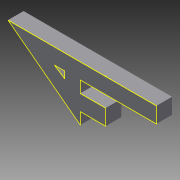
# Autodesk Inventor part: wedger
Saved by Autodesk Inventor 2013 (Build 170138000, 138)
## iProperties
Created: 2013-02-25
Part Number: wedger
Material: Generic
Document SubType Name: Modeling
Designer: Arpan
Density: 1 g/cm^3
Author: Arpan
Autodesk Inventor part; units mm, degrees
ref_plane "YZ Plane" through (0, 0, 0) normal (1, 0, 0) x (0, 1, 0)
ref_plane "XZ Plane" through (0, 0, 0) normal (0, 1, 0) x (-1, 0, 0)
ref_plane "XY Plane" through (0, 0, 0) normal (0, 0, 1) x (1, 0, 0)
sketch "Sketch1" plane through (0, 0, 0) normal (0, 0, 1) x (1, 0, 0)
  line L0 (0, 0) -> (-158.75, 0)
  line L1 (-158.75, 0) -> (-41.275, -88.9)
  line L2 (-41.275, -88.9) -> (-41.275, -25.4)
  line L3 (-41.275, -88.9) -> (-41.275, -69.85)
  line L4 (-41.275, -69.85) -> (0, -69.85)
  line L5 (0, -69.85) -> (0, 0)
  line L6 (-41.275, 0) -> (-66.675, 0)
  line L7 (-66.675, -25.4) -> (-125.1857, -25.4)
  line L8 (-94.622, -48.5293) -> (-79.2945, -28.2752)
  line L9 (-79.2945, -28.2752) -> (-83.0939, -25.4)
  line L10 (-79.2945, -28.2752) -> (-66.675, -37.8251)
  line L11 (-41.275, -69.85) -> (-41.275, -44.45)
  line L12 (-41.275, -44.45) -> (0, -44.45)
  line L13 (0, 0) -> (0, -25.4)
  line L14 (-41.275, -25.4) -> (0, -25.4)
  line L15 (0, -25.4) -> (88.9, -25.4)
  line L16 (88.9, -25.4) -> (88.9, 0)
  line L17 (88.9, 0) -> (0, 0)
  line L18 (-66.675, -25.4) -> (-66.675, -69.6784)
  line L19 (-66.675, -25.4) -> (-41.275, -25.4)
  dimension "d0" = 158.75
  dimension "d1" = 88.9
  dimension "d2" = 41.275
  dimension "d3" = 19.05
  dimension "d5" = 25.4
  dimension "d6" = 25.4
  dimension "d7" = 25.4
  dimension "d8" = 25.4
  dimension "d9" = 88.9
  dimension "d12" = 25.4
  dimension "d13" = 247.65
  dimension "d19" = 142.883
  dimension "d20" = 37.117
  dimension "d21" = 52.883
  dimension "d22" = 147.3214
  dimension "d23" = 42.0918
  constraints: 40 end point, 10 point on line, 8 perpendicular, 3 collinear, 1 horizontal, 1 parallel
  measures "d0" distance of L0.start L0.end
  measures "d1" distance of L1.end L6.start
  measures "d2" distance from line of L0.start L2
  measures "d3" distance of L1.end L3.end
  measures "d5" distance of L7.start L6.end
  measures "d6" distance of L8.start L8.end
  measures "d7" distance of L3.end L11.end
  measures "d8" distance of L2.end L6.start
  measures "d9" distance of L13.end L15.end
  measures "d12" distance between parallel lines of L2 L18
  measures "d13" distance of L16.end L0.end
  measures "d19" angle of L7 L1
  measures "d20" angle of L0 L1
  measures "d21" angle of L2 L1
  measures "d22" distance of L0.end L1.end
  measures "d23" distance of L7.end L0.end
extrude "Extrusion2" add sketch "Sketch1" along normal blind 25.4 contours L5 L14 L19 L7 L1 L0 | L5 L4 L2 L12 | L2 L1 L18 L19 | L7 L9 L8 L1
sketch "Sketch4" plane through (0, 0, 25.4) normal (0, 0, 1) x (1, 0, 0)
  line L0 (0, -25.4) -> (0, 0) projected
  line L1 (0, 0) -> (-158.75, 0) projected
  line L2 (-94.622, -48.5293) -> (-79.2945, -28.2752) projected
  line L3 (-66.675, -25.4) -> (-66.675, -69.6784) projected
  line L4 (-66.675, -69.6784) -> (-41.275, -88.9) projected
  line L5 (-41.275, -88.9) -> (-41.275, -69.85) projected
  line L6 (-79.2945, -28.2752) -> (-66.675, -36.4274)
  line L7 (-94.622, -48.5293) -> (-66.675, -69.6784)
  line L8 (0, -25.4) -> (82.55, -25.4)
  line L9 (82.55, -25.4) -> (82.55, 0)
  line L10 (82.55, 0) -> (0, 0)
  dimension "d16" = 82.55
  constraints: 10 end point, 2 collinear, 2 perpendicular, 1 point on line
  measures "d16" distance of L0.start L8.end
extrude "Extrusion3" add sketch "Sketch4" against normal blind 25.4
sketch "Sketch5" plane through (0, 0, 25.4) normal (0, 0, 1) x (1, 0, 0)
  line L0 (-158.75, 0) -> (-41.275, -88.9) projected
  line L1 (-41.275, -88.9) -> (-41.275, -69.85) projected
  line L2 (-41.275, -69.85) -> (0, -69.85) projected
  line L3 (0, -69.85) -> (0, -44.45) projected
  line L4 (0, -44.45) -> (-41.275, -44.45) projected
  line L5 (-41.275, -44.45) -> (-41.275, -25.4) projected
  line L6 (-41.275, -25.4) -> (82.55, -25.4) projected
  line L7 (82.55, -25.4) -> (82.55, 0) projected
  line L8 (82.55, 0) -> (-158.75, 0) projected
  line L9 (-66.675, -36.4274) -> (-79.2945, -28.2752) projected
  line L10 (-79.2945, -28.2752) -> (-83.0939, -25.4) projected
  line L11 (-83.0939, -25.4) -> (-66.675, -25.4) projected
  line L12 (-66.675, -25.4) -> (-66.675, -36.4274) projected
  point P0 (0, 0)
body "Solid2"
